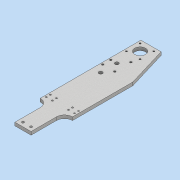
# Autodesk Inventor part: Wspornik pionowy osi Y - prawa strona
Saved by Autodesk Inventor 2018 (Build 220112000, 112)
## iProperties
Created: 2019-01-25
Part Number: Wspornik pionowy osi Y - prawa strona
Material: Ogólny
Document SubType Name: Modeling
Designer: Dawid
Density: 1 g/cm^3
Appearance: Aluminium odlewane
Author: Dawid
Autodesk Inventor part; units mm, degrees
ref_plane "YZ Plane" through (0, 0, 0) normal (1, 0, 0) x (0, 1, 0)
ref_plane "XZ Plane" through (0, 0, 0) normal (0, 1, 0) x (-1, 0, 0)
ref_plane "XY Plane" through (0, 0, 0) normal (0, 0, 1) x (1, 0, 0)
sketch "Szkic1" plane through (0, 0, 0) normal (0, 0, 1) x (1, 0, 0)
  line L0 (0, 0) -> (20, 0)
  line L1 (0, 0) -> (-20, 0)
  line L2 (-20, 0) -> (-20, 20)
  line L3 (-20, 0) -> (0, 0) construction
  line L4 (-20, 20) -> (20, 20)
  line L5 (20, 20) -> (20, 0)
  line L6 (-20, 0) -> (-20, 88)
  line L7 (-20, 88) -> (20, 88)
  line L8 (20, 88) -> (20, 20)
  line L9 (20, 88) -> (20, 93)
  line L10 (20, 93) -> (-20, 93)
  line L11 (-20, 93) -> (-20, 88)
  line L12 (0, 93) -> (35, 93)
  line L13 (35, 93) -> (40, 93)
  line L14 (0, 93) -> (-35, 93)
  line L15 (-35, 93) -> (-40, 93)
  line L16 (-40, 93) -> (-40, 103)
  line L17 (-40, 103) -> (40, 103)
  line L18 (40, 103) -> (40, 93)
  line L19 (-35, 93) -> (-35, 103)
  line L20 (35, 93) -> (35, 103)
  circle A0 centre (-35, 103) radius 1.5
  circle A1 centre (-35, 93) radius 1.5
  circle A2 centre (35, 103) radius 1.5
  circle A3 centre (35, 93) radius 1.5
  line L21 (40, 93) -> (40, 83)
  line L22 (40, 83) -> (20, 83)
  line L23 (-40, 93) -> (-40, 83)
  line L24 (-40, 83) -> (-20, 83)
  line L25 (-40, 103) -> (-40, 183)
  line L26 (40, 103) -> (40, 183)
  line L27 (40, 183) -> (-40, 183)
  dimension "d0" = 20
  dimension "d1" = 20
  dimension "d2" = 20
  dimension "d3" = 90
  dimension "d4" = 88
  dimension "d5" = 5
  dimension "d6" = 35
  dimension "d7" = 5
  dimension "d8" = 35
  dimension "d9" = 5
  dimension "d10" = 10
  dimension "d11" = 3
  dimension "d12" = 3
  dimension "d13" = 3
  dimension "d14" = 3
  dimension "d15" = 10
  dimension "d16" = 10
  dimension "d17" = 80
  dimension "d18" = 80
  constraints: 56 end point, 11 perpendicular, 9 point on line, 6 vertical, 5 horizontal, 4 centre point, 4 coincident, 1 midpoint, 1 parallel
  measures "d0" distance of L0.start L0.end
  measures "d1" distance of L0.start L1.end
  measures "d2" distance of L1.end L2.end
  measures "d3" angle of L3 L2
  measures "d4" distance of L1.end L6.end
  measures "d5" distance of L7.end L9.end
  measures "d6" distance of L12.start L12.end
  measures "d7" distance of L12.end L13.end
  measures "d8" distance of L12.start L14.end
  measures "d9" distance of L14.end L15.end
  measures "d10" distance of L15.end L16.end
  measures "d11" diameter of A0
  measures "d12" diameter of A1
  measures "d13" diameter of A2
  measures "d14" diameter of A3
  measures "d15" distance of L13.end L21.end
  measures "d16" distance of L15.end L23.end
  measures "d17" distance of L16.end L25.end
  measures "d18" distance of L17.end L26.end
extrude "Wyciągnięcie proste1" add sketch "Szkic1" along normal blind 8
sketch "Szkic2" plane through (0, 0, 8) normal (0, 0, 1) x (1, 0, 0)
  circle A0 centre (-35, 103) radius 1.5 projected
  circle A1 centre (-35, 93) radius 1.5 projected
  circle A2 centre (35, 103) radius 1.5 projected
  circle A3 centre (35, 93) radius 1.5 projected
  line L0 (-35, 103) -> (35, 103)
  line L1 (-35, 93) -> (35, 93)
  line L2 (-35, 103) -> (-20, 103)
  line L3 (-20, 103) -> (-20, 93)
  line L4 (35, 103) -> (20, 103)
  line L5 (20, 103) -> (20, 93)
  circle A4 centre (-20, 103) radius 2
  circle A5 centre (-20, 93) radius 2
  circle A6 centre (20, 103) radius 2
  circle A7 centre (20, 93) radius 2
  line L6 (40, 83) -> (40, 183) projected
  line L7 (40, 183) -> (-40, 183) projected
  line L8 (-40, 183) -> (-40, 83) projected
  line L9 (-40, 83) -> (-20, 83) projected
  line L10 (-20, 83) -> (-20, 0) projected
  line L11 (-20, 0) -> (20, 0) projected
  line L12 (20, 0) -> (20, 83) projected
  line L13 (20, 83) -> (40, 83) projected
  line L14 (-20, 0) -> (20, 0) projected
  line L15 (-20, 0) -> (-20, 10)
  line L16 (-20, 83) -> (-20, 0) projected
  line L17 (-20, 10) -> (20, 10)
  line L18 (-20, 10) -> (-10, 10)
  line L19 (20, 10) -> (10, 10)
  circle A8 centre (-10, 10) radius 3
  circle A9 centre (10, 10) radius 3
  point P0 (0, 0)
  dimension "d21" = 15
  dimension "d22" = 15
  dimension "d23" = 4
  dimension "d24" = 4
  dimension "d25" = 4
  dimension "d26" = 4
  dimension "d27" = 10
  dimension "d28" = 10
  dimension "d29" = 10
  dimension "d30" = 6
  dimension "d31" = 6
  constraints: 20 end point, 8 point on line, 6 centre point, 6 coincident, 3 perpendicular, 2 horizontal
  measures "d21" distance of L0.start L2.end
  measures "d22" distance of L0.end L4.end
  measures "d23" diameter of A4
  measures "d24" diameter of A5
  measures "d25" diameter of A6
  measures "d26" diameter of A7
  measures "d27" distance of L10.end L15.end
  measures "d28" distance of L15.end L18.end
  measures "d29" distance of L17.end L19.end
  measures "d30" diameter of A8
  measures "d31" diameter of A9
hole "Otwór1" at (-20, 103, 8) at (-20, 93, 8) at (20, 103, 8) at (20, 93, 8) at (-35, 103, 8) at (-35, 93, 8) at (35, 103, 8) at (35, 93, 8) direction (0, 0, -1) diameter 4 end through all
sketch "Szkic3" plane through (0, 0, 8) normal (0, 0, 1) x (1, 0, 0)
  circle A0 centre (-10, 10) radius 3 projected
  circle A1 centre (10, 10) radius 3 projected
  point P0 (0, 0)
hole "Otwór2" at (-10, 10, 8) at (10, 10, 8) direction (0, 0, -1) diameter 6 end through all
fillet "Zaokrąglenie1" radius 20 2 edges at (20, 83, 4) (-20, 83, 4)
sketch "Szkic4" plane through (0, 0, 8) normal (0, 0, 1) x (1, 0, 0)
  line L0 (40, 183) -> (-40, 183) projected
  line L1 (40, 83) -> (40, 183) projected
  line L2 (40, 183) -> (-40, 183)
  line L3 (-40, 183) -> (-40, 333)
  line L4 (-40, 333) -> (0, 333)
  line L5 (40, 183) -> (40, 233)
  line L6 (40, 233) -> (0, 333)
  point P0 (0, 0)
  dimension "d47" = 150
  dimension "d50" = 50
  constraints: 10 end point, 3 perpendicular, 1 vertical
  measures "d47" distance of L0.end L3.end
  measures "d50" distance of L0.start L5.end
extrude "Wyciągnięcie proste2" add sketch "Szkic4" against normal up to surface (8 mm away)
sketch "Szkic5" plane through (0, 0, 8) normal (0, 0, 1) x (1, 0, 0)
  line L0 (0, 333) -> (-40, 333) projected
  line L1 (-40, 333) -> (-40, 83) projected
  line L2 (-40, 333) -> (-40, 308)
  line L3 (-40, 308) -> (-17, 308)
  circle A0 centre (-17, 308) radius 13.5
  point P0 (0, 0)
  dimension "d51" = 25
  dimension "d52" = 23
  dimension "d53" = 27
  constraints: 4 end point, 1 centre point, 1 coincident, 1 horizontal, 1 point on line
  measures "d51" distance of L0.end L2.end
  measures "d52" distance of L2.end L3.end
  measures "d53" diameter of A0
extrude "Wyciągnięcie proste4" cut sketch "Szkic5" against normal up to next
sketch "Szkic7" plane through (0, 0, 0) normal (0, 0, -1) x (-1, 0, 0)
  line L0 (0, 333) -> (-40, 233) projected
  line L1 (0, 333) -> (40, 333) projected
  line L2 (0, 333) -> (-10, 333)
  line L3 (-10, 333) -> (-40, 233)
  point P0 (0, 0)
  dimension "d59" = 10
  constraints: 4 end point, 1 collinear
  measures "d59" distance of L0.start L2.end
extrude "Wyciągnięcie proste5" add sketch "Szkic7" against normal blind 8
sketch "Szkic9" plane through (0, 0, 0) normal (0, 0, -1) x (-1, 0, 0)
  circle A0 centre (17, 308) radius 15
  line L0 (42, 333) -> (-8, 333)
  line L1 (-8, 333) -> (-23, 283)
  line L2 (-23, 283) -> (42, 283)
  line L3 (42, 283) -> (42, 333)
  line L4 (-10, 333) -> (40, 333) projected
  line L5 (40, 83) -> (40, 333) projected
  circle A1 centre (0, 325) radius 2
  circle A2 centre (34, 325) radius 2
  circle A3 centre (0, 291) radius 2
  circle A4 centre (34, 291) radius 2
  circle A5 centre (17, 308) radius 13.5 projected
  point P0 (0, 0)
  point P1 (42, 283)
  dimension "d62" = 4
  dimension "d63" = 4
  dimension "d64" = 4
  dimension "d65" = 4
  constraints: 8 end point, 5 centre point
  measures "d62" diameter of A1
  measures "d63" diameter of A2
  measures "d64" diameter of A3
  measures "d65" diameter of A4
extrude "Wyciągnięcie proste6" cut sketch "Szkic9" against normal up to next contours A1 | A2 | A3 | A4
thread "Gwint1" size "M4x0.7" class "6H" standard "ANSI Metric M Profile" full length
thread "Gwint2" size "M4x0.7" class "6H" standard "ANSI Metric M Profile" full length
thread "Gwint3" size "M4x0.7" class "6H" standard "ANSI Metric M Profile" full length
thread "Gwint4" size "M4x0.7" class "6H" standard "ANSI Metric M Profile" full length
sketch "Szkic11" plane through (0, 0, 8) normal (0, 0, 1) x (1, 0, 0)
  line L0 (-40, 333) -> (-40, 83) projected
  line L1 (10, 333) -> (-40, 333) projected
  line L2 (-40, 333) -> (-40, 243)
  line L3 (-40, 83) -> (-40, 333) projected
  line L4 (-40, 333) -> (50, 333) construction
  line L5 (-40, 243) -> (0, 243)
  line L6 (0, 243) -> (0, 163)
  line L7 (0, 163) -> (-40, 163)
  line L8 (-40, 243) -> (-20, 243)
  line L9 (-20, 243) -> (-20, 163)
  line L10 (-20, 163) -> (-20, 203)
  line L11 (-20, 243) -> (-20, 223)
  line L12 (-20, 203) -> (-20, 213)
  line L13 (-20, 243) -> (-20, 253)
  circle A0 centre (-20, 213) radius 4.5
  circle A1 centre (-20, 253) radius 4.5
  point P0 (0, 0)
  dimension "d76" = 90
  dimension "d77" = 90
  dimension "d78" = 40
  dimension "d79" = 80
  dimension "d80" = 20
  dimension "d81" = 40
  dimension "d82" = 20
  dimension "d113" = 10
  dimension "d114" = 10
  dimension "d115" = 9
  dimension "d116" = 9
  constraints: 22 end point, 4 coincident, 4 perpendicular, 3 midpoint, 3 point on line, 2 centre point, 1 collinear, 1 horizontal, 1 vertical
  measures "d76" distance of L0.start L2.end
  measures "d77" angle of L2 L4
  measures "d78" distance of L2.end L5.end
  measures "d79" distance of L5.end L6.end
  measures "d80" distance of L2.end L8.end
  measures "d81" distance of L9.end L10.end
  measures "d82" distance of L8.end L11.end
  measures "d113" distance of L12.start L12.end
  measures "d114" distance of L13.start L13.end
  measures "d115" diameter of A0
  measures "d116" diameter of A1
extrude "Wyciągnięcie proste7" cut sketch "Szkic11" against normal up to next contours A1 | A0 L9 | L9 A0
sketch "Szkic12" plane through (0, 0, 8) normal (0, 0, 1) x (1, 0, 0)
  line L0 (40, 233) -> (10, 333)
  line L1 (10, 333) -> (-40, 333)
  line L2 (-40, 333) -> (-40, 83)
  line L3 (40, 83) -> (40, 233)
  arc A0 (-20, 63) -> (-40, 83) centre (-40, 63) ccw
  arc A1 (40, 83) -> (20, 63) centre (40, 63) ccw
  line L4 (-40, 283) -> (20, 283)
  line L5 (20, 283) -> (20, 223)
  line L6 (-40, 223) -> (20, 223)
  line L7 (-40, 223) -> (-40, 283)
  circle A2 centre (0, 291) radius 2 projected
  circle A3 centre (0, 325) radius 2 projected
  circle A4 centre (-34, 325) radius 2 projected
  circle A5 centre (-34, 291) radius 2 projected
  circle A6 centre (-17, 308) radius 13.5 projected
  circle A7 centre (-10, 10) radius 3 projected
  circle A8 centre (10, 10) radius 3 projected
  circle A9 centre (35, 103) radius 2 projected
  circle A10 centre (-35, 103) radius 2 projected
  circle A11 centre (20, 103) radius 2 projected
  circle A12 centre (-20, 103) radius 2 projected
  circle A13 centre (-20, 93) radius 2 projected
  circle A14 centre (20, 93) radius 2 projected
  circle A15 centre (-35, 93) radius 2 projected
  circle A16 centre (35, 93) radius 2 projected
  line L8 (-20, 63) -> (-20, 0) projected
  line L9 (-20, 0) -> (20, 0) projected
  line L10 (20, 0) -> (20, 63) projected
  arc A17 (40, 83) -> (20, 63) centre (40, 63) ccw projected
  line L11 (40, 83) -> (40, 233) projected
  line L12 (40, 233) -> (10, 333) projected
  line L13 (10, 333) -> (-40, 333) projected
  line L14 (-40, 333) -> (-40, 83) projected
  arc A18 (-20, 63) -> (-40, 83) centre (-40, 63) ccw projected
  line L15 (-35, 258) -> (-35, 253)
  line L16 (-5, 278) -> (-5, 273)
  line L17 (-35, 228) -> (-35, 233)
  line L18 (-5, 228) -> (-5, 233)
  circle A19 centre (-35, 233) radius 2.5
  circle A20 centre (-5, 233) radius 2.5
  circle A21 centre (-5, 273) radius 2.5
  circle A22 centre (-35, 253) radius 2.5
  line L19 (-37.5, 248) -> (-37.5, 258)
  arc A23 (-32.5, 258) -> (-37.5, 258) centre (-35, 258) ccw
  line L20 (-32.5, 258) -> (-32.5, 248)
  arc A24 (-37.5, 248) -> (-32.5, 248) centre (-35, 248) ccw
  line L21 (-2.5, 238) -> (-2.5, 228)
  arc A25 (-7.5, 228) -> (-2.5, 228) centre (-5, 228) ccw
  line L22 (-7.5, 228) -> (-7.5, 238)
  arc A26 (-2.5, 238) -> (-7.5, 238) centre (-5, 238) ccw
  line L23 (-37.5, 228) -> (-37.5, 238)
  arc A27 (-32.5, 238) -> (-37.5, 238) centre (-35, 238) ccw
  line L24 (-32.5, 238) -> (-32.5, 228)
  arc A28 (-37.5, 228) -> (-32.5, 228) centre (-35, 228) ccw
  line L25 (-2.5, 278) -> (-2.5, 268)
  arc A29 (-7.5, 268) -> (-2.5, 268) centre (-5, 268) ccw
  line L26 (-7.5, 268) -> (-7.5, 278)
  arc A30 (-2.5, 278) -> (-7.5, 278) centre (-5, 278) ccw
  line L27 (-30, 248) -> (-30, 258)
  arc A31 (-10, 258) -> (-30, 258) centre (-20, 258) ccw
  line L28 (-10, 258) -> (-10, 248)
  arc A32 (-30, 248) -> (-10, 248) centre (-20, 248) ccw
  line L29 (-40, 223) -> (-40, 283)
  line L30 (-40, 223) -> (20, 223)
  line L31 (20, 283) -> (20, 223)
  line L32 (-40, 283) -> (20, 283)
  line L33 (-35, 278) -> (-35, 283)
  line L34 (-5, 278) -> (-5, 283)
  line L35 (-35, 228) -> (-35, 223)
  line L36 (-5, 228) -> (-5, 223)
  line L37 (10, 333) -> (-40, 333) projected
  line L38 (-40, 333) -> (-40, 283)
  line L39 (-40, 83) -> (-40, 333) projected
  point P0 (0, 0)
  point P1 (30, 43)
  point P2 (-35, 248)
  point P3 (-5, 268)
  point P4 (-5, 238)
  point P5 (-35, 238)
  dimension "d87" = 5
  dimension "d88" = 5
  dimension "d89" = 5
  dimension "d90" = 5
  dimension "d91" = 5
  dimension "d92" = 5
  dimension "d93" = 5
  dimension "d94" = 5
  dimension "d118" = 50
  constraints: 62 end point, 24 point on circle, 16 centre point, 5 point on line, 4 coincident, 3 perpendicular, 2 other
  measures "d87" distance of L15.start L15.end
  measures "d88" distance of L16.start L16.end
  measures "d89" distance of L17.start L17.end
  measures "d90" distance of L18.start L18.end
  measures "d91" diameter of A19
  measures "d92" diameter of A20
  measures "d93" diameter of A21
  measures "d94" diameter of A22
  measures "d118" distance of L1.end L38.end
extrude "Wyciągnięcie proste8" cut sketch "Szkic12" against normal up to next contours A19 | A21 | A20 | A22
thread "Gwint9" size "M4x0.7" class "6H" standard "ANSI Metric M Profile" full length
thread "Gwint10" size "M4x0.7" class "6H" standard "ANSI Metric M Profile" full length
thread "Gwint11" size "M4x0.7" class "6H" standard "ANSI Metric M Profile" full length
thread "Gwint12" size "M4x0.7" class "6H" standard "ANSI Metric M Profile" full length
thread "Gwint13" size "M5x0.8" class "6H" standard "ANSI Metric M Profile" full length
thread "Gwint14" size "M5x0.8" class "6H" standard "ANSI Metric M Profile" full length
thread "Gwint15" size "M5x0.8" class "6H" standard "ANSI Metric M Profile" full length
thread "Gwint16" size "M5x0.8" class "6H" standard "ANSI Metric M Profile" full length
